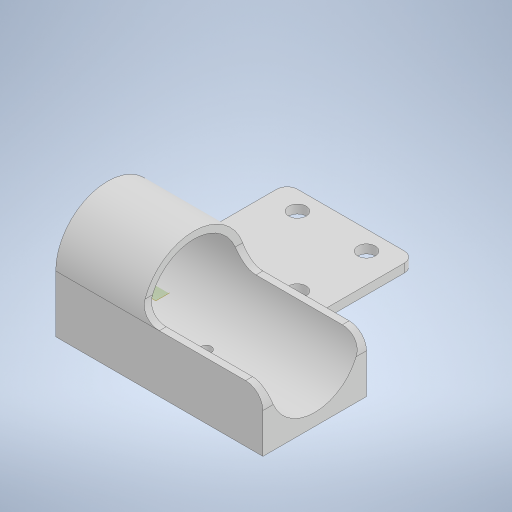
# Autodesk Inventor part: myMotorHolder
Saved by Autodesk Inventor 2023.1 (Build 271208000, 208)
## iProperties
Created: 2025-08-13
Part Number: myMotorHolder
Material: Типовые
Document SubType Name: Modeling
Designer: DELL
Density: 1 g/cm^3
Appearance: По умолчанию
Author: DELL
Autodesk Inventor part; units mm, degrees
ref_plane "YZ Plane" through (0, 0, 0) normal (1, 0, 0) x (0, 1, 0)
ref_plane "XZ Plane" through (0, 0, 0) normal (0, 1, 0) x (-1, 0, 0)
ref_plane "XY Plane" through (0, 0, 0) normal (0, 0, 1) x (1, 0, 0)
sketch "Эскиз1" plane through (0, 0, 0) normal (1, 0, 0) x (0, 1, 0)
  circle A0 centre (0, 0) radius 13
  circle A1 centre (0, 0) radius 15
  line L0 (0, -15) -> (-15, -15)
  line L1 (-15, -15) -> (-15, 15)
  line L2 (-15, 15) -> (0, 15)
  point P0 (-15, 0)
  dimension "d0" = 26
  dimension "d1" = 30
  constraints: 6 end point, 2 centre point, 2 coincident, 2 perpendicular, 2 point on circle, 2 tangent, 1 horizontal
  measures "d0" diameter of A0
  measures "d1" diameter of A1
extrude "Выдавливание1" add sketch "Эскиз1" along normal blind 60 contours A0 | A1 | A1 L1 L2 | L0 L1 A1
sketch "Эскиз2" plane through (60, 0, 0) normal (1, 0, 0) x (0, 0, 1)
  circle A0 centre (0, 0) radius 13
  dimension "d4" = 26
  constraints: 1 centre point, 1 coincident
  measures "d4" diameter of A0
extrude "Выдавливание2" cut sketch "Эскиз2" against normal blind 57
sketch "Эскиз3" plane through (0, 0, 0) normal (-1, 0, 0) x (0, 0, -1)
  circle A0 centre (0, 0) radius 3.6
  circle A1 centre (8.5, 0) radius 1.55
  circle A2 centre (-8.5, 0) radius 1.55
  line L0 (-8.5, 0) -> (8.5, 0) construction
  dimension "d7" = 7.2
  dimension "d8" = 3.1
  dimension "d9" = 3.1
  dimension "d10" = 17
  constraints: 3 centre point, 2 coincident, 2 end point, 1 horizontal, 1 midpoint
  measures "d7" diameter of A0
  measures "d8" diameter of A1
  measures "d9" diameter of A2
  measures "d10" distance of L0.start L0.end
extrude "Выдавливание3" cut sketch "Эскиз3" against normal blind 3
chamfer "Фаска1" distance 1.65 angle 45 2 edges at (0, 0, 10.05) (0, 0, -6.95)
sketch "Эскиз7" plane through (60, 0, 0) normal (1, 0, 0) x (0, 0, -1)
  arc A0 (15, 0) -> (-15, 0) centre (0, 0) ccw projected
  line L0 (-15, 0) -> (17, 0)
  line L1 (17, 0) -> (17, 16)
  line L2 (17, 16) -> (-15, 16)
  line L3 (-15, 16) -> (-15, 0)
  point P0 (15, 0)
  dimension "d25" = 32
  dimension "d26" = 16
  constraints: 8 end point, 2 parallel, 1 horizontal, 1 perpendicular
  measures "d25" distance of L2.end L1.end
  measures "d26" distance of L1.end L0.end
extrude "Выдавливание5" cut sketch "Эскиз7" against normal blind 35 contours L0 A0
fillet "Сопряжение1" radius 5 4 edges at (25, 0, 14) (25, 0, -14) (60, 0, -14) (60, 0, 14)
ref_plane "РабПлоскость5" through (0, -11, -14) normal (0, -1, 0) x (1, 0, 0)
sketch "Эскиз14" plane through (0, -15, -15) normal (0, 0, -1) x (-1, 0, 0)
  line L0 (0, 1) -> (-60, 1)
  line L1 (-60, 1) -> (-60, 3.5)
  line L2 (-60, 3.5) -> (0, 3.5)
  line L3 (0, 3.5) -> (0, 1)
  line L4 (0, 0) -> (0, 15) projected
  line L5 (0, 0) -> (-60, 0) projected
  dimension "d66" = 60
  dimension "d67" = 2.5
  dimension "d68" = 1
  constraints: 8 end point, 2 parallel, 1 horizontal, 1 perpendicular, 1 point on line
  measures "d66" distance of L1.end L2.end
  measures "d67" distance of L0.end L1.end
  measures "d68" distance between parallel lines of L5 L0
extrude "Выдавливание11" add sketch "Эскиз14" along normal blind 37
sketch "Эскиз15" plane through (0, -15, -15) normal (0, -1, 0) x (1, 0, 0)
  line L0 (60, 30) -> (60, 0) projected
  line L1 (0, 0) -> (60, 0)
  line L2 (60, 0) -> (60, 30)
  line L3 (60, 30) -> (0, 30)
  line L4 (0, 30) -> (0, 0)
  dimension "d76" = 30
  constraints: 8 end point, 2 parallel, 1 horizontal, 1 perpendicular
  measures "d76" distance of L3.end L1.start
extrude "Выдавливание12" add sketch "Эскиз15" along normal blind 1.5
sketch "Эскиз16" plane through (60, 0, 0) normal (1, 0, 0) x (0, 0, -1)
  line L0 (15, -14) -> (52, -14) projected
  line L1 (15, -11.5) -> (52, -11.5) projected
  line L2 (15, -14) -> (52, -14)
  line L3 (52, -14) -> (52, -11.5)
  line L4 (52, -11.5) -> (15, -11.5)
  line L5 (15, -11.5) -> (15, -14)
  point P0 (0, 0)
  constraints: 8 end point, 2 parallel, 1 horizontal, 1 perpendicular
extrude "Выдавливание13" cut sketch "Эскиз16" against normal blind 23
fillet "Сопряжение4" radius 3 4 edges at (37, -12.75, -52) (0, -12.75, -52) (18.5, -11.5, -15) (37, -12.75, -15)
sketch "Эскиз12" plane through (0, -11, -14) normal (0, -1, 0) x (1, 0, 0)
  circle A0 centre (28.5, 14) radius 1.55
  line L0 (0, 29) -> (60, 29) projected
  point P0 (0, 14)
  dimension "d56" = 3.1
  dimension "d65" = 15
  constraints: 1 centre point
  measures "d56" diameter of A0
  measures "d65" distance from line of L0 A0.centre
extrude "Выдавливание10" cut sketch "Эскиз12" along normal mid plane 35
sketch "Эскиз17" plane through (0, -11.5, -18) normal (0, 1, 0) x (1, 0, 0)
  circle A0 centre (8.5, 28.5) radius 2.55 projected
  circle A1 centre (28.5, 28.5) radius 2.55 projected
  circle A2 centre (8.5, 8.5) radius 2.55 projected
  circle A3 centre (28.5, 8.5) radius 2.55 projected
  point P0 (0, -18)
extrude "Выдавливание14" cut sketch "Эскиз17" against normal blind 23
